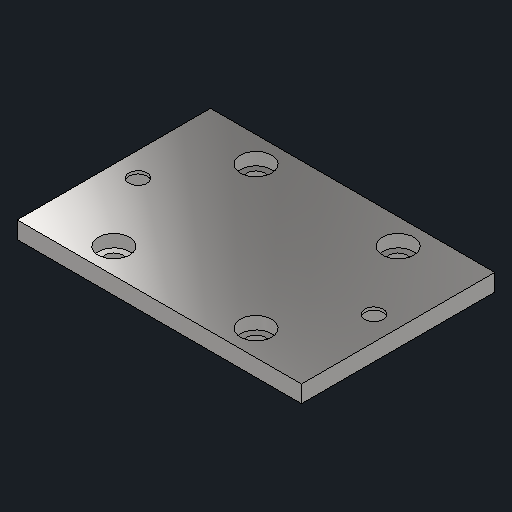
# Autodesk Inventor part: KN-00-01-02
Saved by Autodesk Inventor 2025.2 (Build 292293000, 293)
## iProperties
Created: 2025-04-24
Part Number: KN-00-01-02
Material: X5CrNi18-10
Document SubType Name: Modeling
Designer: Kacper Mik
Density: 8 g/cm^3
Appearance: Semi-Polished
Mass: 404.06 g
Surface Area: 173.913 cm^2
Volume: 50.5075 cm^3
Author: Kacper Mik
Autodesk Inventor part; units mm, degrees
ref_plane "YZ Plane" through (0, 0, 0) normal (1, 0, 0) x (0, 1, 0)
ref_plane "XZ Plane" through (0, 0, 0) normal (0, 1, 0) x (-1, 0, 0)
ref_plane "XY Plane" through (0, 0, 0) normal (0, 0, 1) x (1, 0, 0)
sketch "Sketch1" plane through (0, 0, 0) normal (0, 1, 0) x (-1, 0, 0)
  line L0 (-50, 34) -> (50, 34)
  line L1 (50, 34) -> (50, -34)
  line L2 (50, -34) -> (-50, -34)
  line L3 (-50, -34) -> (-50, 34)
  line L4 (-50, 34) -> (50, -34) construction
  line L5 (50, 34) -> (-50, -34) construction
  point P0 (0, 0)
  dimension "d0" = 68
  dimension "d1" = 100
  constraints: 12 end point, 2 midpoint, 2 parallel, 1 horizontal, 1 perpendicular
  measures "d0" distance of L0.end L1.end
  measures "d1" distance of L1.end L2.end
extrude "Extrusion1" add sketch "Sketch1" along normal blind 6
sketch "Sketch2" plane through (0, 0, 0) normal (0, 1, 0) x (1, 0, 0)
  line L0 (0, 47.6) -> (0, -47.6) projected
  point P0 (0, 0)
  point P1 (-41.5, 0)
  point P2 (41.5, 0)
  dimension "d4" = 83
  constraints: 2 horizontal alignment, 1 symmetric about line
  measures "d4" distance of point (41.5, 0) point (-41.5, 0)
sketch "Sketch3" plane through (0, 6, 0) normal (0, 1, 0) x (1, 0, 0)
  line L0 (25, 25) -> (-25, 25) construction
  line L1 (-25, 25) -> (-25, -25) construction
  line L2 (-25, -25) -> (25, -25) construction
  line L3 (25, -25) -> (25, 25) construction
  line L4 (25, 25) -> (-25, -25) construction
  line L5 (-25, 25) -> (25, -25) construction
  point P0 (0, 0)
  dimension "d12" = 50
  dimension "d13" = 50
  constraints: 12 end point, 4 coincident, 2 midpoint, 2 parallel, 1 horizontal, 1 perpendicular
  measures "d12" distance of L2.end L1.end
  measures "d13" distance of L1.end L0.end
hole "Hole2" at (-25, 6, 25) at (-25, 6, -25) at (25, 6, -25) at (25, 6, 25) direction (0, -1, 0) diameter 6.6 end through all counterbore diameter 11 counterbore depth 4.4 clearance for "Socket Head Cap Screw ISO 4762" size "M6" standard "ISO"
hole "Hole3" at (-41.5, 0, 0) at (41.5, 0, 0) direction (0, 1, 0) diameter 6.4 end through all counterbore diameter 11 counterbore depth 5 clearance for "Socket Head Cap Screw ISO 4762" size "M6" standard "ISO"
body "Solid1"
